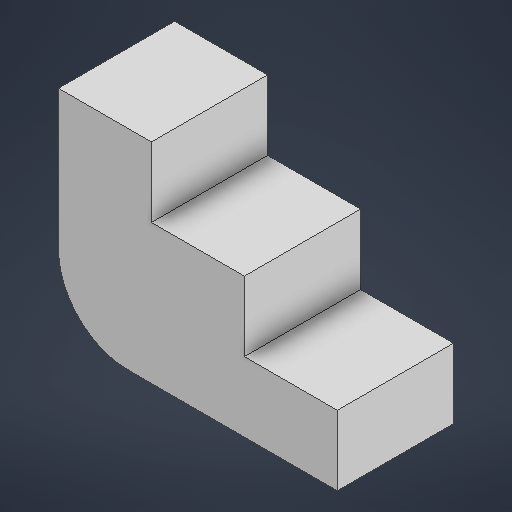
# Autodesk Inventor part: Part5
Saved by Autodesk Inventor 2026 (Build 300175050, 175E)
## iProperties
Created: 2026-03-19
Part Number: Part5
Material: Generic
Document SubType Name: Modeling
Designer: Administrator
Density: 1 g/cm^3
Appearance: Default
Author: Administrator
Autodesk Inventor part; units mm, degrees
ref_plane "YZ Plane" through (0, 0, 0) normal (1, 0, 0) x (0, 1, 0)
ref_plane "XZ Plane" through (0, 0, 0) normal (0, 1, 0) x (-1, 0, 0)
ref_plane "XY Plane" through (0, 0, 0) normal (0, 0, 1) x (1, 0, 0)
sketch "Sketch1" plane through (0, 0, 0) normal (0, 0, 1) x (1, 0, 0)
  line L0 (0, 0) -> (60, 0)
  line L1 (60, 0) -> (60, 15)
  line L2 (60, 15) -> (40, 15)
  line L3 (40, 15) -> (40, 30)
  line L4 (40, 30) -> (20, 30)
  line L5 (20, 30) -> (20, 45)
  line L6 (20, 45) -> (0, 45)
  line L7 (0, 45) -> (0, 0)
  dimension "d0" = 15
  dimension "d2" = 20
  dimension "d3" = 45
  dimension "d4" = 60
  dimension "d5" = 20
  dimension "d10" = 15
  constraints: 16 end point, 7 perpendicular, 1 horizontal
  measures "d0" distance of L0.end L1.end
  measures "d2" distance of L5.end L6.end
  measures "d3" distance of L6.end L0.start
  measures "d4" distance of L0.start L0.end
  measures "d5" distance of L3.end L4.end
  measures "d10" distance of L2.end L3.end
extrude "Extrusion1" add sketch "Sketch1" along normal mid plane 25
fillet "Fillet1" radius 15 1 edges at (0, 0, 0)
body "Solid1"
